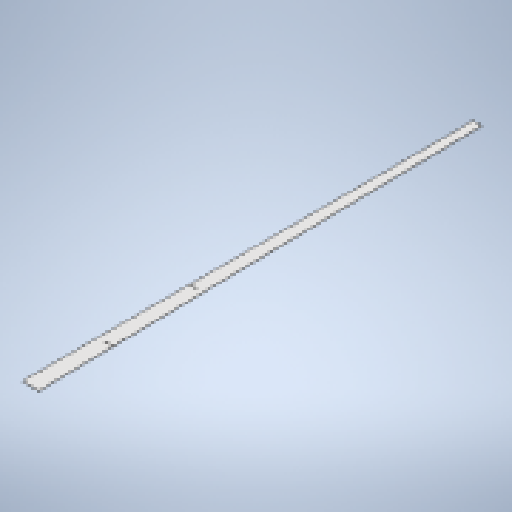
# Autodesk Inventor part: BSH 022 rib 2
Saved by Autodesk Inventor 2025 (Build 290162010, 162A)
## iProperties
Created: 2024-07-23
Part Number: BSH 022 rib 2
Material: Stainless Steel
Document SubType Name: Sheet Metal
Designer: admin
Density: 8 g/cm^3
Sheet Metal Rule: AISI304 3mm Die 32
Appearance: Default
Author: admin
Autodesk Inventor part; units mm, degrees
ref_plane "YZ Plane" through (0, 0, 0) normal (1, 0, 0) x (0, 1, 0)
ref_plane "XZ Plane" through (0, 0, 0) normal (0, 1, 0) x (-1, 0, 0)
ref_plane "XY Plane" through (0, 0, 0) normal (0, 0, 1) x (1, 0, 0)
sketch "Sketch1" plane through (0, 0, 0) normal (0, 0, 1) x (1, 0, 0)
  line L0 (1200, 2950) -> (-1200, 2950)
  line L1 (-1200, 2950) -> (-1200, 0)
  line L2 (-1200, 0) -> (1200, 0)
  line L3 (1200, 0) -> (1200, 2950)
  line L4 (1150, 2950) -> (1150, 0)
  line L5 (-1150, 0) -> (-1150, 2950) construction
  line L6 (0, 2950) -> (0, 50) construction
  line L7 (-1100, 200) -> (-950, 50)
  line L8 (-1200, 100) -> (-1100, 100)
  line L9 (-1100, 100) -> (-1100, 0)
  line L10 (-1100, 200) -> (-1150, 2950)
  arc A0 (-1100.4545, 224.9959) -> (-1082.3223, 182.3223) centre (-1100, 200) ccw
  arc A1 (-1082.3223, 182.3223) -> (-1100.4545, 224.9959) centre (-1100, 200) ccw construction
  line L11 (-1200, 255) -> (-1101, 255)
  line L12 (0, 50) -> (-950, 50)
  line L13 (0, 50) -> (0, 0)
  line L14 (1505.3449, -225.894) -> (355.3449, -225.894)
  dimension "d3" = 2400
  dimension "d4" = 2950
  dimension "d5" = 50
  dimension "d6" = 100
  dimension "d7" = 50
  dimension "d8" = 2695
  dimension "d9" = 135
  dimension "d10" = 950
  dimension "d11" = 1150
  dimension "d12" = 136.042
  dimension "d13" = 50
  dimension "d14" = 100
  dimension "d15" = 212.132
  dimension "d17" = 55
  dimension "d20" = 200
  measures "d3" distance of L3.start L1.end
  measures "d4" distance of L1.end L1.start
  measures "d5" diameter of A0
  measures "d6" distance of L8.start L8.end
  measures "d7" distance between parallel lines of L1 L5
  measures "d8" distance between parallel lines of L0 L11
  measures "d9" angle of L12 L7
  measures "d10" distance of L6.end L7.end
  measures "d11" distance of L14.start L14.end
  measures "d12" angle of L7 L10
  measures "d13" distance between parallel lines of L2 L12
  measures "d14" distance from line of L1 L10.start
  measures "d15" distance of L10.start L7.end
  measures "d17" vertical distance of L10.start L11.end
  measures "d20" distance from line of L2 A1.centre
extrude "Plate1" add sketch "Sketch1" along normal blind 3 contours L10 L11 L1 L0
sketch "Sketch2" plane through (0, 0, 3) normal (0, 0, 1) x (1, 0, 0)
  line L0 (-1101, 255) -> (-1200, 255) projected
  line L1 (-1150, 2950) -> (-1101, 255) projected
  line L2 (-1200, 2950) -> (-1150, 2950) projected
  line L3 (-1200, 255) -> (-1200, 2950) projected
  line L4 (-1101, 255) -> (-1150, 2950) projected
  line L5 (-1109.2386, 708.1251) -> (-1155.6482, 707.2813)
  line L6 (-1155.6482, 707.2813) -> (-1155.5901, 704.0818)
  line L7 (-1155.5901, 704.0818) -> (-1109.1805, 704.9256)
  line L8 (-1119.4188, 1268.0326) -> (-1158.7385, 1267.3177) construction
  line L9 (-1158.7385, 1267.3177) -> (-1158.6803, 1264.1182)
  line L10 (-1158.6803, 1264.1182) -> (-1119.3606, 1264.8331) construction
  line L11 (-1150, 2950) -> (-1101, 255) projected
  line L12 (-1158.6803, 1264.1182) -> (-1200, 1263.3669)
  line L13 (-1158.7385, 1267.3177) -> (-1200, 1266.5675)
  point P0 (0, 0)
  point P1 (-1119.3606, 1264.8331)
  dimension "d21" = 3.2
  dimension "d22" = 46.4173
  dimension "d23" = 450
  dimension "d24" = 3.2
  dimension "d28" = 560
  dimension "d31" = 41.3197
  constraints: 16 end point, 6 point on line, 5 perpendicular, 2 collinear, 1 parallel
  measures "d21" distance of L5.end L6.end
  measures "d22" distance of L6.end L7.end
  measures "d23" distance of L0.start L7.end
  measures "d24" distance of L8.end L9.end
  measures "d28" distance of L5.start L8.start
  measures "d31" horizontal distance of L12.end L9.end
extrude "Extrusion1" cut sketch "Sketch2" against normal through all contours L7 L6 L5 L1 | L3 L13 L9 L12
equation "\"d11\" = d10 + d18"
equation "\"d14\" = d6"
equation "\"d23\" = Stringer1_hight"
equation "\"d28\" = Stringer1_step"
equation "\"d2\" = Thickness"
equation "\"BendReliefWidth\" = Thickness"
equation "\"BendReliefDepth\" = 0.5 * Thickness"
equation "\"CornerReliefSize\" = 4 * Thickness"
equation "\"MinimumRemnant\" = 2 * Thickness"
equation "\"TransitionRadius\" = BendRadius"
equation "\"JacobiRadiusSize\" = BendRadius"
equation "\"GapSize\" = Thickness"
equation "\"d18\" = d19"
equation "\"Stringer1_hight\" = 450"
equation "\"Stringer1_step\" = 560"
equation "\"Thickness\" = 3"
equation "\"BendRadius\" = 5"
equation "\"d19\" = 200"
body "Solid1"
